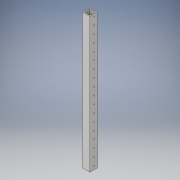
# Autodesk Inventor part: lil silver hangy thing
Saved by Autodesk Inventor 2018 (Build 220112000, 112)
## iProperties
Created: 2018-02-12
Part Number: lil silver hangy thing
Material: Generic
Document SubType Name: Sheet Metal
Designer: cruz.anthony
Density: 1 g/cm^3
Sheet Metal Rule: Default
Appearance: Default
Author: cruz.anthony
Autodesk Inventor part; units mm, degrees
ref_plane "YZ Plane" through (0, 0, 0) normal (1, 0, 0) x (0, 1, 0)
ref_plane "XZ Plane" through (0, 0, 0) normal (0, 1, 0) x (-1, 0, 0)
ref_plane "XY Plane" through (0, 0, 0) normal (0, 0, 1) x (1, 0, 0)
sketch "Sketch1" plane through (0, 0, 0) normal (0, 1, 0) x (-1, 0, 0)
  line L0 (0, 0) -> (25.4, 0)
  line L1 (25.4, 0) -> (25.4, -25.4)
  line L2 (25.4, -25.4) -> (0, -25.4)
  line L3 (0, -25.4) -> (0, 0)
  dimension "d0" = 25.4
  dimension "d1" = 25.4
  constraints: 8 end point, 2 parallel, 1 horizontal, 1 perpendicular
  measures "d0" distance of L1.end L2.end
  measures "d1" distance of L0.end L1.end
extrude "Extrusion1" add sketch "Sketch1" along normal blind 450.85
sketch "Sketch2" plane through (0, 450.85, 0) normal (0, 1, 0) x (1, 0, 0)
  line L0 (-3.175, 3.175) -> (-22.225, 3.175)
  line L1 (-22.225, 3.175) -> (-22.225, 22.225)
  line L2 (-22.225, 22.225) -> (-3.175, 22.225)
  line L3 (-3.175, 22.225) -> (-3.175, 3.175)
  line L4 (0, 25.4) -> (-25.4, 25.4) projected
  line L5 (-25.4, 25.4) -> (-25.4, 0) projected
  line L6 (-25.4, 0) -> (0, 0) projected
  line L7 (0, 0) -> (0, 25.4) projected
  dimension "d4" = 3.175
  dimension "d5" = 3.175
  dimension "d6" = 3.175
  dimension "d7" = 3.175
  constraints: 8 end point, 2 parallel, 1 horizontal, 1 perpendicular
  measures "d4" distance between parallel lines of L4 L2
  measures "d5" distance between parallel lines of L5 L1
  measures "d6" distance between parallel lines of L6 L0
  measures "d7" distance between parallel lines of L7 L3
extrude "Extrusion2" cut sketch "Sketch2" against normal blind 450.85 contours L0 L1 L2 L3
sketch "Sketch3" plane through (-25.4, 0, -25.4) normal (-1, 0, 0) x (0, 0, 1)
  circle A0 centre (12.7, 12.7) radius 1.4605
  line L0 (0, 0) -> (0, 450.85) projected
  line L1 (25.4, 0) -> (0, 0) projected
  circle A1 centre (12.7, 38.1) radius 1.4605
  circle A2 centre (12.7, 63.5) radius 1.4605
  circle A3 centre (12.7, 88.9) radius 1.4605
  circle A4 centre (12.7, 114.3) radius 1.4605
  circle A5 centre (12.7, 139.7) radius 1.4605
  circle A6 centre (12.7, 165.1) radius 1.4605
  circle A7 centre (12.7, 190.5) radius 1.4605
  circle A8 centre (12.7, 215.9) radius 1.4605
  circle A9 centre (12.7, 241.3) radius 1.4605
  circle A10 centre (12.7, 266.7) radius 1.4605
  circle A11 centre (12.7, 292.1) radius 1.4605
  circle A12 centre (12.7, 317.5) radius 1.4605
  circle A13 centre (12.7, 342.9) radius 1.4605
  circle A14 centre (12.7, 368.3) radius 1.4605
  circle A15 centre (12.7, 393.7) radius 1.4605
  circle A16 centre (12.7, 419.1) radius 1.4605
  circle A17 centre (12.7, 444.5) radius 1.4605
  dimension "d10" = 2.921
  dimension "d11" = 12.7
  dimension "d12" = 12.7
  dimension "d15" = 25.4
  constraints: 18 centre point, 1 vertical, 34 other
  measures "d10" diameter of A0
  measures "d11" distance from line of L0 A0.centre
  measures "d12" distance from line of L1 A0.centre
  measures "d15" distance of A0.centre A1.centre
extrude "Extrusion3" cut sketch "Sketch3" against normal blind 25.4
equation "\"BendRadius\" = Thickness"
equation "\"BendReliefWidth\" = Thickness"
equation "\"BendReliefDepth\" = 0.5 * Thickness"
equation "\"CornerReliefSize\" = 4 * Thickness"
equation "\"MinimumRemnant\" = 2 * Thickness"
equation "\"TransitionRadius\" = BendRadius"
equation "\"JacobiRadiusSize\" = BendRadius"
equation "\"GapSize\" = Thickness"
equation "\"Thickness\" = 3.048"
body "Solid1"
